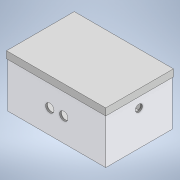
# Autodesk Inventor part: cajaEléctrica
Saved by Autodesk Inventor 2020 (Build 240168000, 168)
## iProperties
Created: 2021-10-16
Part Number: cajaEléctrica
Material: Genérico
Document SubType Name: Modeling
Designer: DANIEL
Density: 1 g/cm^3
Appearance: Valor por defecto
Author: DANIEL
Autodesk Inventor part; units mm, degrees
ref_plane "YZ Plane" through (0, 0, 0) normal (1, 0, 0) x (0, 1, 0)
ref_plane "XZ Plane" through (0, 0, 0) normal (0, 1, 0) x (-1, 0, 0)
ref_plane "XY Plane" through (0, 0, 0) normal (0, 0, 1) x (1, 0, 0)
sketch "Boceto1" plane through (0, 0, 0) normal (0, 1, 0) x (-1, 0, 0)
  line L0 (140, 95) -> (-140, 95)
  line L1 (-140, 95) -> (-140, -95)
  line L2 (-140, -95) -> (140, -95)
  line L3 (140, -95) -> (140, 95)
  point P0 (0, 0)
  dimension "d0" = 280
  dimension "d1" = 190
  dimension "d2" = 95
  dimension "d3" = 140
  constraints: 8 end point, 2 parallel, 1 horizontal, 1 perpendicular
  measures "d0" distance between parallel lines of L1 L3
  measures "d1" distance between parallel lines of L2 L0
  measures "d2" distance from line of L0 point (0, 0)
  measures "d3" distance from line of point (0, 0) L1
extrude "Extrusión1" add sketch "Boceto1" along normal blind 130
ref_plane "Plano de trabajo1" through (0, 0, 95) normal (1, 0, 0) x (0, 0, -1)
ref_plane "Plano de trabajo2" through (140, 0, 0) normal (0, 0, -1) x (-1, 0, 0)
sketch "Boceto3" plane through (0, 130, 0) normal (0, 1, 0) x (1, 0, 0)
  line L0 (140, 95) -> (-140, 95) projected
  line L1 (-140, 95) -> (-140, -95) projected
  line L2 (-140, -95) -> (140, -95) projected
  line L3 (140, -95) -> (140, 95) projected
  line L4 (-135, -90) -> (135, -90)
  line L5 (135, -90) -> (135, 90)
  line L6 (135, 90) -> (-135, 90)
  line L7 (-135, 90) -> (-135, -90)
  point P0 (0, 0)
  dimension "d7" = 270
  dimension "d8" = 135
  dimension "d9" = 180
  dimension "d10" = 90
  constraints: 8 end point, 2 parallel, 1 horizontal, 1 perpendicular
  measures "d7" distance between parallel lines of L5 L7
  measures "d8" distance from line of L7 point (0, 0)
  measures "d9" distance between parallel lines of L6 L4
  measures "d10" distance from line of L4 point (0, 0)
extrude "Extrusión2" cut sketch "Boceto3" against normal blind 125 contours L7 L6 L5 L4
sketch "Boceto4" plane through (-140, 0, -95) normal (-1, 0, 0) x (0, 0, 1)
  circle A0 centre (95, 29.1709) radius 10
  point P0 (95, 0)
  dimension "d13" = 20
  constraints: 1 centre point
  measures "d13" diameter of A0
extrude "Extrusión3" [suppressed]
sketch "Boceto7" plane through (-140, 0, 95) normal (0, 0, 1) x (1, 0, 0)
  circle A0 centre (140, 68) radius 10
  line L0 (0, 0) -> (280, 0) projected
  line L1 (280, 0) -> (280, 130) projected
  point P0 (140, 0)
  dimension "d18" = 20
  dimension "d19" = 68
  dimension "d20" = 140
  constraints: 1 centre point
  measures "d18" diameter of A0
  measures "d19" distance from line of A0.centre L0
  measures "d20" distance from line of A0.centre L1
extrude "Extrusión5" [suppressed]
sketch "Boceto8" plane through (0, 130, 0) normal (0, 1, 0) x (1, 0, 0)
  line L0 (-142, 97) -> (142, 97)
  line L1 (142, 97) -> (142, -97)
  line L2 (142, -97) -> (-142, -97)
  line L3 (-142, -97) -> (-142, 97)
  line L4 (140, 95) -> (-140, 95) projected
  line L5 (140, -95) -> (140, 95) projected
  line L6 (-140, -95) -> (140, -95) projected
  line L7 (-140, 95) -> (-140, -95) projected
  point P0 (0, 0)
  dimension "d23" = 2
  dimension "d24" = 2
  dimension "d25" = 2
  dimension "d26" = 2
  constraints: 8 end point, 2 parallel, 1 horizontal, 1 perpendicular
  measures "d23" distance between parallel lines of L3 L7
  measures "d24" distance between parallel lines of L0 L4
  measures "d25" distance between parallel lines of L1 L5
  measures "d26" distance between parallel lines of L6 L2
extrude "Techo" add sketch "Boceto8" along normal blind 20 contours L0 L1 L2 L3 | L5 L6 L7 L4
sketch "Boceto9" plane through (-140, 0, 95) normal (0, 0, 1) x (1, 0, 0)
  circle A0 centre (120, 68) radius 12
  circle A1 centre (160, 68) radius 12
  circle A2 centre (140, 68) radius 10 projected
  line L0 (0, 0) -> (280, 0) projected
  line L1 (0, 0) -> (0, 130) projected
  point P0 (140, 0)
  point P1 (148.9, 63.4404)
  point P2 (148.9, 72.5596)
  point P3 (131.1, 63.4404)
  point P4 (131.1, 72.5596)
  dimension "d29" = 24
  dimension "d30" = 24
  dimension "d31" = 68
  dimension "d32" = 40
  dimension "Q" = 120
  constraints: 2 centre point, 1 horizontal alignment
  measures "d29" diameter of A0
  measures "d30" diameter of A1
  measures "d31" distance from line of L0 A0.centre
  measures "d32" distance of A0.centre A1.centre
  measures "Q" distance from line of L1 A0.centre
extrude "Extrusión7" cut sketch "Boceto9" against normal blind 10 contours A0 A2 | A2 A0 | A2 A1 | A1 A2
sketch "Boceto10" plane through (140, 0, 95) normal (1, 0, 0) x (0, 0, -1)
  circle A0 centre (95, 100) radius 10.15
  line L0 (0, 0) -> (0, 130) projected
  line L1 (0, 130) -> (190, 130) projected
  point P0 (95, 0)
  dimension "d36" = 20.3
  dimension "d37" = 95
  dimension "d38" = 30
  constraints: 1 centre point
  measures "d36" diameter of A0
  measures "d37" distance from line of L0 A0.centre
  measures "d38" distance from line of L1 A0.centre
extrude "Extrusión8" cut sketch "Boceto10" against normal blind 10
sketch "Boceto11" plane through (-140, 0, -95) normal (-1, 0, 0) x (0, 0, 1)
  line L0 (0, 130) -> (190, 130) projected
  circle A0 centre (95, 70) radius 4.5
  line L1 (0, 0) -> (0, 130) projected
  point P0 (95, 0)
  dimension "d45" = 9
  dimension "d46" = 60
  dimension "d47" = 95
  constraints: 1 centre point
  measures "d45" diameter of A0
  measures "d46" distance from line of L0 A0.centre
  measures "d47" distance from line of L1 A0.centre
extrude "Extrusión10" cut sketch "Boceto11" against normal blind 10
